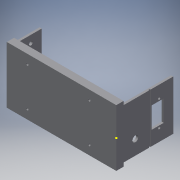
# Autodesk Inventor part: box
Saved by Autodesk Inventor 2018 (Build 220112000, 112)
## iProperties
Created: 2018-05-21
Part Number: box
Material: Generic
Document SubType Name: Modeling
Designer: David
Density: 1 g/cm^3
Appearance: Default
Author: David
Autodesk Inventor part; units mm, degrees
ref_plane "YZ Plane" through (0, 0, 0) normal (1, 0, 0) x (0, 1, 0)
ref_plane "XZ Plane" through (0, 0, 0) normal (0, 1, 0) x (-1, 0, 0)
ref_plane "XY Plane" through (0, 0, 0) normal (0, 0, 1) x (1, 0, 0)
sketch "Sketch1" plane through (0, 0, 0) normal (0, 1, 0) x (-1, 0, 0)
  line L0 (-75, -39) -> (75, -39)
  line L1 (75, -39) -> (75, 39)
  line L2 (75, 39) -> (-75, 39)
  line L3 (-75, 39) -> (-75, -39)
  line L4 (-75, -39) -> (75, 39) construction
  line L5 (75, -39) -> (-75, 39) construction
  point P0 (0, 0)
  dimension "d0" = 150
  dimension "d1" = 78
  constraints: 12 end point, 2 midpoint, 2 parallel, 1 horizontal, 1 perpendicular
  measures "d0" distance of L2.end L1.end
  measures "d1" distance of L1.end L0.end
extrude "Extrusion1" add sketch "Sketch1" along normal blind 45
sketch "Sketch4" plane through (75, 0, 39) normal (1, 0, 0) x (0, 0, -1)
  line L0 (78, 45) -> (0, 45) projected
  line L1 (0, 45) -> (5, 45)
  line L2 (5, 45) -> (5, 10)
  line L3 (5, 10) -> (0, 10)
  line L4 (0, 10) -> (0, 45)
  line L5 (78, 45) -> (73, 45)
  line L6 (73, 45) -> (73, 10)
  line L7 (73, 10) -> (78, 10)
  line L8 (78, 10) -> (78, 45)
  point P0 (39, 0)
  dimension "d14" = 5
  dimension "d15" = 35
  dimension "d16" = 5
  dimension "d17" = 35
  constraints: 16 end point, 4 parallel, 2 horizontal, 2 perpendicular
  measures "d14" distance of L2.end L3.end
  measures "d15" distance of L1.end L2.end
  measures "d16" distance of L7.end L6.end
  measures "d17" distance of L6.end L5.end
extrude "Extrusion4" cut sketch "Sketch4" against normal blind 150
sketch "Sketch5" plane through (0, 45, 0) normal (0, 1, 0) x (1, 0, 0)
  line L0 (72, 36) -> (-72, 36)
  line L1 (-72, 36) -> (-72, -36)
  line L2 (-72, -36) -> (72, -36)
  line L3 (72, -36) -> (72, 36)
  line L4 (72, 36) -> (-72, -36) construction
  line L5 (-72, 36) -> (72, -36) construction
  point P0 (0, 0)
  dimension "d20" = 144
  dimension "d21" = 72
  constraints: 12 end point, 2 midpoint, 2 parallel, 1 horizontal, 1 perpendicular
  measures "d20" distance of L2.end L1.end
  measures "d21" distance of L1.end L0.end
extrude "Extrusion5" cut sketch "Sketch5" against normal blind 42
sketch "Sketch6" plane through (75, 0, 39) normal (1, 0, 0) x (0, 0, -1)
  circle A0 centre (53, 26.1062) radius 4
  line L0 (73, 10) -> (73, 45) projected
  circle A1 centre (25, 27.5) radius 10.75
  line L1 (5, 78) -> (5, 10) projected
  point P0 (39, 0)
  point P1 (5, 45)
  dimension "d25" = 8
  dimension "d33" = 20
  dimension "d67" = 21.5
  dimension "d68" = 20
  constraints: 2 centre point
  measures "d25" diameter of A0
  measures "d33" distance from line of L0 A0.centre
  measures "d67" diameter of A1
  measures "d68" distance from line of L1 A1.centre
sketch "Sketch7" plane through (-75, 0, -39) normal (-1, 0, 0) x (0, 0, 1)
  line L0 (22.15, 28.0506) -> (22.15, 31.9494)
  line L1 (15.05, 31.9494) -> (15.05, 28.0506)
  line L2 (15.05, 28.0506) -> (22.15, 31.9494) construction
  line L3 (22.15, 28.0506) -> (15.05, 31.9494) construction
  arc A0 (22.15, 31.9494) -> (15.05, 31.9494) centre (18.6, 30) ccw
  arc A1 (15.05, 28.0506) -> (22.15, 28.0506) centre (18.6, 30) ccw
  line L4 (18.6, 30) -> (18, 30) construction
  line L5 (0, 0) -> (78, 0) projected
  line L6 (5, 45) -> (5, 10) projected
  arc A2 (20.8062, 10.85) -> (16.3938, 10.85) centre (18.6, 15) ccw
  line L7 (16.3938, 10.85) -> (20.8062, 10.85)
  circle A3 centre (32.2, 30) radius 2.5
  line L8 (49.35, 28.0506) -> (49.35, 31.9494)
  line L9 (42.25, 31.9494) -> (42.25, 28.0506)
  line L10 (42.25, 28.0506) -> (49.35, 31.9494) construction
  line L11 (49.35, 28.0506) -> (42.25, 31.9494) construction
  arc A4 (49.35, 31.9494) -> (42.25, 31.9494) centre (45.8, 30) ccw
  arc A5 (42.25, 28.0506) -> (49.35, 28.0506) centre (45.8, 30) ccw
  line L12 (45.8, 30) -> (41.8, 30) construction
  line L13 (43.5938, 10.85) -> (48.0062, 10.85)
  arc A6 (48.0062, 10.85) -> (43.5938, 10.85) centre (45.8, 15) ccw
  circle A7 centre (62.8, 30) radius 2.5
  point P0 (39, 0)
  point P1 (18.6, 30)
  point P2 (18.6, 30)
  dimension "d36" = 7.1
  dimension "d37" = 4.05
  dimension "d77" = 30
  dimension "d81" = 13.6
  dimension "d85" = 9.4
  dimension "d86" = 4.15
  dimension "d87" = 15
  dimension "d88" = 5
  dimension "d89" = 13.6
  dimension "d90" = 7.1
  dimension "d91" = 4.05
  dimension "d92" = 9.4
  dimension "d93" = 4.15
  dimension "d94" = 15
  dimension "d95" = 5
  dimension "d96" = 17
  dimension "d97" = 13.6
  constraints: 24 end point, 12 point on circle, 8 centre point, 8 midpoint, 4 horizontal, 3 horizontal alignment, 2 parallel, 2 vertical, 2 vertical alignment
  measures "d36" distance between parallel lines of L0 L1
  measures "d37" radius of A1
  measures "d77" distance between parallel lines of L5 L4
  measures "d81" distance from line of L6 L4.start
  measures "d85" diameter of A2
  measures "d86" distance from line of L7 A2.centre
  measures "d87" distance of L4.start A2.centre
  measures "d88" diameter of A3
  measures "d89" distance of A3.centre L4.start
  measures "d90" distance between parallel lines of L8 L9
  measures "d91" radius of A5
  measures "d92" diameter of A6
  measures "d93" distance from line of L13 A6.centre
  measures "d94" distance of L12.start A6.centre
  measures "d95" diameter of A7
  measures "d96" distance of A7.centre L12.start
  measures "d97" distance of L12.start A3.centre
sketch "Sketch8" plane through (0, 3, 0) normal (0, 1, 0) x (1, 0, 0)
  line L0 (-47, -26.5) -> (38, -26.5)
  line L1 (38, -26.5) -> (38, 26.5)
  line L2 (38, 26.5) -> (-47, 26.5)
  line L3 (-47, 26.5) -> (-47, -26.5)
  line L4 (-47, -26.5) -> (38, 26.5) construction
  line L5 (38, -26.5) -> (-47, 26.5) construction
  circle A0 centre (38, 26.5) radius 1.6
  circle A1 centre (38, -26.5) radius 1.6
  circle A2 centre (-47, -26.5) radius 1.6
  circle A3 centre (-47, 26.5) radius 1.6
  line L6 (-72, -34) -> (-72, 34) projected
  point P0 (-4.5, 0)
  dimension "d42" = 85
  dimension "d43" = 53
  dimension "d44" = 3.2
  dimension "d45" = 3.2
  dimension "d46" = 3.2
  dimension "d47" = 3.2
  dimension "d51" = 25
  constraints: 12 end point, 4 centre point, 4 coincident, 2 midpoint, 2 parallel, 1 horizontal, 1 perpendicular
  measures "d42" distance of L2.end L1.end
  measures "d43" distance of L1.end L0.end
  measures "d44" diameter of A0
  measures "d45" diameter of A1
  measures "d46" diameter of A2
  measures "d47" diameter of A3
  measures "d51" distance between parallel lines of L6 L3
extrude "Extrusion8" cut sketch "Sketch8" against normal blind 3 contours L3 A2 L0 | L0 A2 L3 | A1 L1 L0 | L0 L1 A1 | A3 L2 L3 | L3 L2 A3 | A0 L2 L1 | L1 L2 A0
sketch "Sketch9" plane through (0, 45, 0) normal (0, 1, 0) x (1, 0, 0)
  line L0 (75, -34) -> (72, -34) projected
  line L1 (75, 39) -> (75, 34) projected
  line L2 (72, -34) -> (75, -34)
  line L3 (75, -34) -> (75, 34)
  line L4 (75, 34) -> (72, 34)
  line L5 (72, 34) -> (72, -34)
  point P0 (0, 0)
  constraints: 8 end point, 2 parallel, 1 horizontal, 1 perpendicular
extrude "Extrusion9" add sketch "Sketch9" along normal blind 33
sketch "Sketch10" plane through (75, 0, 39) normal (1, 0, 0) x (0, 0, -1)
  line L0 (53.5, 65) -> (24.5, 65)
  line L1 (24.5, 65) -> (24.5, 48.5)
  line L2 (24.5, 48.5) -> (53.5, 48.5)
  line L3 (53.5, 48.5) -> (53.5, 65)
  line L4 (53.5, 65) -> (24.5, 48.5) construction
  line L5 (24.5, 65) -> (53.5, 48.5) construction
  line L6 (61.5, 65) -> (16.5, 65)
  line L7 (16.5, 65) -> (16.5, 48.5)
  line L8 (16.5, 48.5) -> (61.5, 48.5)
  line L9 (61.5, 48.5) -> (61.5, 65)
  line L10 (61.5, 65) -> (16.5, 48.5) construction
  line L11 (16.5, 65) -> (61.5, 48.5) construction
  line L12 (39, 48.5) -> (39, 65) construction
  line L13 (5, 78) -> (73, 78) projected
  line L14 (5, 78) -> (5, 10) projected
  circle A0 centre (21.5, 59) radius 1.6
  line L15 (39, 65) -> (39, 48.5)
  circle A1 centre (56.5, 59) radius 1.6
  point P0 (39, 0)
  point P1 (39, 56.75)
  point P2 (39, 56.75)
  dimension "d54" = 29
  dimension "d55" = 16.5
  dimension "d56" = 45
  dimension "d59" = 13
  dimension "d60" = 34
  dimension "d61" = 3.2
  dimension "d62" = 5
  dimension "d74" = 10.5
  constraints: 28 end point, 7 midpoint, 4 parallel, 3 perpendicular, 2 centre point, 2 horizontal, 1 point on line, 1 symmetric about line, 1 other
  measures "d54" distance of L2.end L1.end
  measures "d55" distance of L1.end L1.start
  measures "d56" distance of L11.end L7.end
  measures "d59" distance between parallel lines of L13 L0
  measures "d60" distance from line of L14 point (39, 56.75)
  measures "d61" diameter of A0
  measures "d62" distance from line of A0.centre L7
  measures "d74" distance from line of L8 A1.centre
extrude "Extrusion10" cut sketch "Sketch10" against normal blind 3 contours L3 L2 L15 L0 | L15 L2 L1 L0 | A0 | A1
sketch "Sketch11" plane through (75, 0, 39) normal (1, 0, 0) x (0, 0, -1)
  point P0 (39, 0)
sketch "Sketch12" plane through (75, 0, 39) normal (1, 0, 0) x (0, 0, -1)
  line L0 (5, 78) -> (5, 10) projected
  line L1 (5, 45) -> (73, 45)
  line L2 (73, 45) -> (73, 47)
  line L3 (73, 47) -> (5, 47)
  line L4 (5, 47) -> (5, 45)
  line L5 (0, 0) -> (78, 0) projected
  line L6 (73, 10) -> (73, 78) projected
  point P0 (39, 0)
  dimension "d69" = 45
  dimension "d70" = 2
  constraints: 8 end point, 2 parallel, 1 collinear, 1 horizontal, 1 perpendicular, 1 point on line
  measures "d69" distance between parallel lines of L5 L1
  measures "d70" distance of L1.end L2.end
extrude "Extrusion12" cut sketch "Sketch12" against normal blind 1
extrude "Extrusion13" cut sketch "Sketch6" against normal blind 10 contours A0
extrude "Extrusion14" cut sketch "Sketch7" against normal blind 10
body "Solid1"
